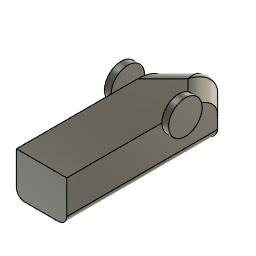
DuckHead v5 (Autodesk Fusion 360 design; units mm, degrees)
Autodesk Fusion 360 part; units mm, degrees
note: some values were not read from the file. Set by a fixed rule: which sketch regions a step uses.
sketch "Sketch1" plane through (0, 0, 0) normal (0, 0, 1) x (1, 0, 0)
sketch "Sketch2" plane through (0, 0, 0) normal (0, 0, 1) x (1, 0, 0)
sketch "Sketch3" plane through (0, 0, 0) normal (0, 0, 1) x (1, 0, 0)
  line L0 (0, 0) -> (0, 50)
  line L1 (0, 50) -> (15, 65)
  line L2 (15, 65) -> (30, 50)
  line L3 (30, 50) -> (30, 0)
  line L4 (30, 0) -> (0, 0)
  constraint coincident L0.start L4.end
  constraint vertical L0
  constraint perpendicular L1 L2
  constraint parallel L0 L3
  constraint perpendicular L0 L4
extrude "Extrude1" add sketch "Sketch3" along normal blind 25
fillet "Fillet1" radius 12.5 2 edges at (22.5, 57.5, 25) (7.5, 57.5, 25)
fillet "Fillet2" radius 5 4 edges at (0, 25, 0) (30, 25, 0) (22.5, 57.5, 0) (7.5, 57.5, 0)
fillet "Fillet3" radius 5 3 edges at (15, 62.9289, 1.4645) (15, 65, 8.75) (15, 59.8223, 21.3388)
extrude "Extrude2" add 1 faces at (11.6667, 0, 16.6667) along direction (0, -1, 0) blind 40
extrude "Extrude3" cut 1 faces at (26.1785, 53.8215, 7.5) along direction (-0.707107, -0.707107, 0) blind 2
extrude "Extrude4" cut 1 faces at (3.8215, 53.8215, 7.5) along direction (0.707107, -0.707107, 0) blind 2
sketch "Sketch4" plane through (0, 0, 0) normal (-1, 0, 0) x (0, -1, 0)
  line L0 (-50, 5) -> (40, 5)
  line L1 (40, 5) -> (40, 25)
  line L2 (40, 25) -> (-32.3223, 25)
  ellipse E0 centre (-32.3223, 12.5) end of major axis (-50, 12.5) minor radius 12.5 (-32.3223, 25) -> (-50, 12.5) ccw
  line L3 (-50, 12.5) -> (-50, 5)
  circle A0 centre (-26.4534, 25) radius 10
  dimension "d15" = 20
  constraint coincident L2 A0.centre
  measures "d15" diameter of A0
extrude "Extrude5" add sketch "Sketch4" along normal blind 3 contours L2 E0 A0 | L2 E0 A0
extrude "Extrude6" add 1 faces at (-3, 25.7282, 28.0287) along direction (-1, 0, 0) blind 1
sketch "Sketch5" plane through (30, 0, 0) normal (1, 0, 0) x (0, 1, 0)
  line L0 (-40, 5) -> (50, 5)
  line L1 (50, 5) -> (50, 12.5)
  ellipse E0 centre (32.3223, 12.5) end of major axis (50, 12.5) minor radius 12.5 (50, 12.5) -> (32.3223, 25) ccw
  line L2 (32.3223, 25) -> (-40, 25)
  line L3 (-40, 25) -> (-40, 5)
  circle A0 centre (26.7382, 25) radius 10
  dimension "d20" = 20
  constraint coincident L2 A0.centre
  measures "d20" diameter of A0
extrude "Extrude7" add sketch "Sketch5" along normal blind 4 contours E0 L2 A0 | E0 L2 A0
